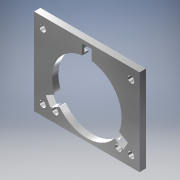
# Autodesk Inventor part: trackball_base
Saved by Autodesk Inventor 2018 (Build 220112000, 112)
## iProperties
Created: 2018-04-03
Part Number: trackball_base
Material: アルミニウム 6061
Document SubType Name: Modeling
Designer: NaMACHAN
Density: 2.7 g/cm^3
Appearance: アルミニウム - フラット
Author: NaMACHAN
Autodesk Inventor part; units mm, degrees
ref_plane "YZ Plane" through (0, 0, 0) normal (1, 0, 0) x (0, 1, 0)
ref_plane "XZ Plane" through (0, 0, 0) normal (0, 1, 0) x (-1, 0, 0)
ref_plane "XY Plane" through (0, 0, 0) normal (0, 0, 1) x (1, 0, 0)
sketch "スケッチ1" plane through (0, 0, 0) normal (0, 1, 0) x (-1, 0, 0)
  line L0 (-25, -16.9) -> (25, -16.9)
  line L1 (25, -16.9) -> (25, 23)
  line L2 (25, 23) -> (-25, 23)
  line L3 (-25, 23) -> (-25, -16.9)
  point P0 (0, 0)
  point P1 (0, 23)
  dimension "d0" = 50
  dimension "d62" = 23
  dimension "d63" = 16.9
  constraints: 8 end point, 2 parallel, 1 horizontal, 1 midpoint, 1 perpendicular, 1 vertical alignment
  measures "d0" distance of L2.end L1.end
  measures "d62" distance from line of L2 point (0, 0)
  measures "d63" distance from line of L0 point (0, 0)
extrude "押し出し1" add sketch "スケッチ1" along normal blind 3
sketch "スケッチ2" plane through (0, 3, 0) normal (0, 1, 0) x (1, 0, 0)
  circle A0 centre (0, 0) radius 16.5
  dimension "d4" = 33
  constraints: 1 centre point, 1 coincident
  measures "d4" diameter of A0
extrude "押し出し2" cut sketch "スケッチ2" against normal blind 3
sketch "スケッチ3" plane through (0, 3, 0) normal (0, 1, 0) x (1, 0, 0)
  line L0 (-6, -17) -> (6, -17)
  line L1 (6, -17) -> (6, -19)
  line L2 (6, -19) -> (-6, -19)
  line L3 (-6, -19) -> (-6, -17)
  line L4 (-6, -17) -> (6, -19) construction
  line L5 (6, -17) -> (-6, -19) construction
  line L6 (-13.4545, 14.6962) -> (-19.4545, 4.3038)
  line L7 (-19.4545, 4.3038) -> (-17.7224, 3.3038)
  line L8 (-17.7224, 3.3038) -> (-11.7224, 13.6962)
  line L9 (-11.7224, 13.6962) -> (-13.4545, 14.6962)
  line L10 (-13.4545, 14.6962) -> (-17.7224, 3.3038) construction
  line L11 (-19.4545, 4.3038) -> (-11.7224, 13.6962) construction
  line L12 (-25, 16.9) -> (-25, -23) projected
  line L13 (11.7224, 13.6962) -> (17.7224, 3.3038)
  line L14 (17.7224, 3.3038) -> (19.4545, 4.3038)
  line L15 (19.4545, 4.3038) -> (13.4545, 14.6962)
  line L16 (13.4545, 14.6962) -> (11.7224, 13.6962)
  line L17 (11.7224, 13.6962) -> (19.4545, 4.3038) construction
  line L18 (17.7224, 3.3038) -> (13.4545, 14.6962) construction
  line L19 (25, -23) -> (25, 16.9) projected
  point P0 (0, 0)
  point P1 (0, -18)
  point P2 (-15.5885, 9)
  point P3 (15.5885, 9)
  point P4 (15.5885, 9)
  point P5 (15.5885, 9)
  dimension "d7" = 120
  dimension "d8" = 120
  dimension "d9" = 18
  dimension "d10" = 18
  dimension "d11" = 18
  dimension "d12" = 2
  dimension "d13" = 12
  dimension "d14" = 30
  dimension "d15" = 12
  dimension "d16" = 2
  dimension "d17" = 30
  dimension "d18" = 2
  dimension "d19" = 12
  constraints: 36 end point, 7 midpoint, 6 parallel, 3 perpendicular, 1 coincident, 1 horizontal, 1 vertical alignment
  measures "d9" distance of point (0, 0) point (0, -18)
  measures "d10" distance of point (-15.588, 9) point (0, 0)
  measures "d11" distance of point (15.588, 9) point (0, 0)
  measures "d12" distance of L0.end L1.end
  measures "d13" distance between parallel lines of L1 L3
  measures "d14" angle of L12 L6
  measures "d15" distance of L7.end L8.end
  measures "d16" distance of L6.end L7.end
  measures "d17" angle of L19 L15
  measures "d18" distance of L15.end L13.start
  measures "d19" distance of L13.start L13.end
extrude "押し出し3" cut sketch "スケッチ3" against normal blind 2
sketch "スケッチ4" plane through (0, 3, 0) normal (0, 1, 0) x (1, 0, 0)
  line L0 (2.25, -14.75) -> (2.25, -21.25)
  line L1 (2.25, -21.25) -> (-2.25, -21.25)
  line L2 (-2.25, -21.25) -> (-2.25, -14.75)
  line L3 (-2.25, -14.75) -> (2.25, -14.75)
  line L4 (2.25, -14.75) -> (-2.25, -21.25) construction
  line L5 (2.25, -21.25) -> (-2.25, -14.75) construction
  line L6 (17.278, 12.5736) -> (11.6489, 9.3236)
  line L7 (11.6489, 9.3236) -> (13.8989, 5.4264)
  line L8 (13.8989, 5.4264) -> (19.528, 8.6764)
  line L9 (19.528, 8.6764) -> (17.278, 12.5736)
  line L10 (17.278, 12.5736) -> (13.8989, 5.4264) construction
  line L11 (11.6489, 9.3236) -> (19.528, 8.6764) construction
  line L12 (25, -23) -> (25, 16.9) projected
  line L13 (-17.278, 12.5736) -> (-11.6489, 9.3236)
  line L14 (-11.6489, 9.3236) -> (-13.8989, 5.4264)
  line L15 (-13.8989, 5.4264) -> (-19.528, 8.6764)
  line L16 (-19.528, 8.6764) -> (-17.278, 12.5736)
  line L17 (-17.278, 12.5736) -> (-13.8989, 5.4264) construction
  line L18 (-11.6489, 9.3236) -> (-19.528, 8.6764) construction
  line L19 (-25, 16.9) -> (-25, -23) projected
  point P0 (0, 0)
  point P1 (15.5885, 9)
  point P2 (0, -18)
  point P3 (-15.5885, 9)
  dimension "d28" = 120
  dimension "d29" = 120
  dimension "d30" = 18
  dimension "d31" = 18
  dimension "d32" = 18
  dimension "d33" = 30
  dimension "d34" = 6.5
  dimension "d35" = 4.5
  dimension "d38" = 6.5
  dimension "d39" = 4.5
  dimension "d40" = 4.5
  dimension "d41" = 6.5
  dimension "d42" = 30
  constraints: 36 end point, 6 midpoint, 6 parallel, 3 perpendicular, 1 vertical, 1 vertical alignment
  measures "d30" distance of point (0, 0) point (0, -18)
  measures "d31" distance of point (-15.588, 9) point (0, 0)
  measures "d32" distance of point (15.588, 9) point (0, 0)
  measures "d33" angle of L12 L9
  measures "d34" distance of L6.start L6.end
  measures "d35" distance of L6.end L7.end
  measures "d38" distance of L1.end L2.end
  measures "d39" distance of L2.end L0.start
  measures "d40" distance of L15.end L13.start
  measures "d41" distance of L14.end L15.end
  measures "d42" angle of L19 L16
extrude "押し出し4" cut sketch "スケッチ4" against normal blind 3
sketch "スケッチ5" plane through (0, 3, 0) normal (0, 1, 0) x (1, 0, 0)
  line L0 (-25, -23) -> (25, -23) projected
  line L1 (25, 16.9) -> (-25, 16.9) projected
  line L2 (-25, 16.9) -> (-25, -23) projected
  line L3 (25, -23) -> (25, 16.9) projected
  point P0 (0, 0)
  point P1 (21, -18)
  point P2 (-21, -18)
  point P3 (-21, 2)
  point P4 (21, 2)
  point P5 (15, 2)
  point P6 (-15, 2)
  dimension "d45" = 5
  dimension "d48" = 5
  dimension "d49" = 4
  dimension "d50" = 4
  dimension "d51" = 4
  dimension "d52" = 4
  dimension "d60" = 6
  dimension "d61" = 6
  dimension "d64" = 20
  constraints: 3 horizontal alignment
  measures "d45" distance from line of L0 point (21, -18)
  measures "d48" distance from line of L0 point (-21, -18)
  measures "d49" distance from line of L2 point (-21, -18)
  measures "d50" distance from line of point (-21, 2) L2
  measures "d51" distance from line of L3 point (21, 2)
  measures "d52" distance from line of L3 point (21, -18)
  measures "d60" distance of point (-21, 2) point (-15, 2)
  measures "d61" distance of point (21, 2) point (15, 2)
  measures "d64" distance of point (21, 2) point (21, -18)
hole "穴1" at (21, 3, 18) at (-21, 3, 18) at (-21, 3, -2) at (21, 3, -2) at (15, 3, -2) at (-15, 3, -2) direction (0, -1, 0) diameter 3 end through all
